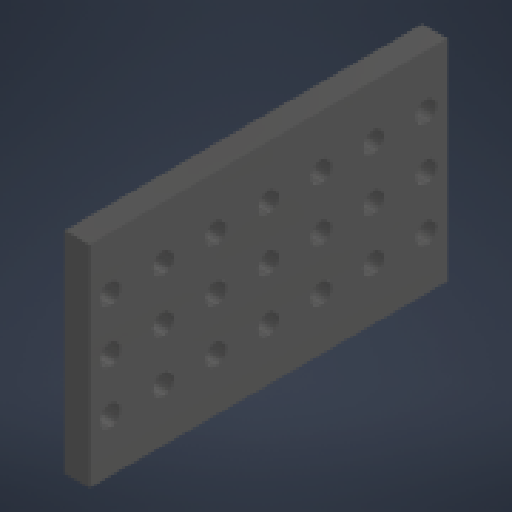
# Autodesk Inventor part: CHAPA FIXAÇÃO ESQUERDA 1
Saved by Autodesk Inventor 2026 (Build 300175000, 175)
## iProperties
Created: 2026-06-17
Part Number: CHAPA FIXAÇÃO ESQUERDA 1
Material: Genérico
Document SubType Name: Modeling
Designer: DELL
Density: 1 g/cm^3
Appearance: Cinza escuro
Author: DELL
Autodesk Inventor part; units mm, degrees
ref_plane "YZ Plane" through (0, 0, 0) normal (1, 0, 0) x (0, 1, 0)
ref_plane "XZ Plane" through (0, 0, 0) normal (0, 1, 0) x (-1, 0, 0)
ref_plane "XY Plane" through (0, 0, 0) normal (0, 0, 1) x (1, 0, 0)
sketch "Esboço1" plane through (0, 0, 0) normal (1, 0, 0) x (0, 1, 0)
  line L0 (0, 0) -> (50.8, 0)
  line L1 (50.8, 0) -> (50.8, -86.2)
  line L2 (50.8, -86.2) -> (0, -86.2)
  line L3 (0, -86.2) -> (0, 0)
  dimension "d0" = 50.8
  dimension "d1" = 86.2
  constraints: 8 end point, 2 parallel, 1 horizontal, 1 perpendicular
  measures "d0" distance of L1.end L2.end
  measures "d1" distance of L0.end L1.end
extrude "Extrusão1" add sketch "Esboço1" along normal blind 6
sketch "Esboço2" plane through (6, 0, 0) normal (1, 0, 0) x (0, 0, -1)
  circle A0 centre (5, 12.7) radius 2.5
  circle A1 centre (5, 25.4) radius 2.5
  circle A2 centre (5, 38.1) radius 2.5
  line L0 (0, 50.8) -> (0, 0) projected
  line L1 (86.2, 50.8) -> (0, 50.8) projected
  line L2 (0, 0) -> (86.2, 0) projected
  dimension "d4" = 5
  dimension "d5" = 5
  dimension "d6" = 5
  dimension "d7" = 5
  dimension "d8" = 5
  dimension "d9" = 5
  dimension "d10" = 12.7
  dimension "d11" = 12.7
  dimension "d12" = 12.7
  constraints: 3 centre point
  measures "d4" diameter of A0
  measures "d5" diameter of A1
  measures "d6" diameter of A2
  measures "d7" distance from line of L0 A0.centre
  measures "d8" distance from line of L0 A1.centre
  measures "d9" distance from line of L0 A2.centre
  measures "d10" distance from line of L1 A2.centre
  measures "d11" distance of A2.centre A1.centre
  measures "d12" distance of A1.centre A0.centre
extrude "Extrusão2" cut sketch "Esboço2" against normal blind 6
pattern_linear "Padrão retangular1" count 7 spacing 12.7 along (0, 0, -1) of "Extrusão2"
sketch "Esboço4" plane through (0, 0, 0) normal (-1, 0, 0) x (0, 0, 1)
  line L0 (-86.2, 0) -> (-86.2, 50.8) projected
  line L1 (-86.2, 50.8) -> (-162.4, 50.8)
  line L2 (-162.4, 50.8) -> (-162.4, 0)
  line L3 (-162.4, 0) -> (-86.2, 0)
  line L4 (-86.2, 0) -> (-86.2, 50.8)
  circle A0 centre (-157.4, 38.1) radius 2.5 projected
  circle A1 centre (-157.4, 25.4) radius 2.5 projected
  circle A2 centre (-157.4, 12.7) radius 2.5 projected
  circle A3 centre (-144.7, 12.7) radius 2.5 projected
  circle A4 centre (-144.7, 25.4) radius 2.5 projected
  circle A5 centre (-144.7, 38.1) radius 2.5 projected
  circle A6 centre (-132, 38.1) radius 2.5 projected
  circle A7 centre (-132, 25.4) radius 2.5 projected
  circle A8 centre (-132, 12.7) radius 2.5 projected
  line L5 (0, 0) -> (0, 50.8) projected
  line L6 (0, 50.8) -> (-467.2, 50.8) projected
  line L7 (-467.2, 50.8) -> (-467.2, 0) projected
  line L8 (0, 0) -> (-467.2, 0) projected
  circle A9 centre (-462.2, 12.7) radius 2.5 projected
  circle A10 centre (-462.2, 25.4) radius 2.5 projected
  circle A11 centre (-462.2, 38.1) radius 2.5 projected
  circle A12 centre (-449.5, 12.7) radius 2.5 projected
  circle A13 centre (-449.5, 25.4) radius 2.5 projected
  circle A14 centre (-449.5, 38.1) radius 2.5 projected
  circle A15 centre (-436.8, 12.7) radius 2.5 projected
  circle A16 centre (-436.8, 25.4) radius 2.5 projected
  circle A17 centre (-436.8, 38.1) radius 2.5 projected
  circle A18 centre (-424.1, 12.7) radius 2.5 projected
  circle A19 centre (-424.1, 25.4) radius 2.5 projected
  circle A20 centre (-424.1, 38.1) radius 2.5 projected
  circle A21 centre (-411.4, 12.7) radius 2.5 projected
  circle A22 centre (-411.4, 25.4) radius 2.5 projected
  circle A23 centre (-411.4, 38.1) radius 2.5 projected
  circle A24 centre (-398.7, 12.7) radius 2.5 projected
  circle A25 centre (-398.7, 25.4) radius 2.5 projected
  circle A26 centre (-398.7, 38.1) radius 2.5 projected
  circle A27 centre (-386, 12.7) radius 2.5 projected
  circle A28 centre (-386, 25.4) radius 2.5 projected
  circle A29 centre (-386, 38.1) radius 2.5 projected
  circle A30 centre (-373.3, 12.7) radius 2.5 projected
  circle A31 centre (-373.3, 25.4) radius 2.5 projected
  circle A32 centre (-373.3, 38.1) radius 2.5 projected
  circle A33 centre (-360.6, 12.7) radius 2.5 projected
  circle A34 centre (-360.6, 25.4) radius 2.5 projected
  circle A35 centre (-360.6, 38.1) radius 2.5 projected
  circle A36 centre (-347.9, 12.7) radius 2.5 projected
  circle A37 centre (-347.9, 25.4) radius 2.5 projected
  circle A38 centre (-347.9, 38.1) radius 2.5 projected
  circle A39 centre (-335.2, 12.7) radius 2.5 projected
  circle A40 centre (-335.2, 25.4) radius 2.5 projected
  circle A41 centre (-335.2, 38.1) radius 2.5 projected
  circle A42 centre (-322.5, 12.7) radius 2.5 projected
  circle A43 centre (-322.5, 25.4) radius 2.5 projected
  circle A44 centre (-322.5, 38.1) radius 2.5 projected
  circle A45 centre (-309.8, 12.7) radius 2.5 projected
  circle A46 centre (-309.8, 25.4) radius 2.5 projected
  circle A47 centre (-309.8, 38.1) radius 2.5 projected
  circle A48 centre (-297.1, 12.7) radius 2.5 projected
  circle A49 centre (-297.1, 25.4) radius 2.5 projected
  circle A50 centre (-297.1, 38.1) radius 2.5 projected
  circle A51 centre (-284.4, 12.7) radius 2.5 projected
  circle A52 centre (-284.4, 25.4) radius 2.5 projected
  circle A53 centre (-284.4, 38.1) radius 2.5 projected
  circle A54 centre (-271.7, 12.7) radius 2.5 projected
  circle A55 centre (-271.7, 25.4) radius 2.5 projected
  circle A56 centre (-271.7, 38.1) radius 2.5 projected
  circle A57 centre (-259, 12.7) radius 2.5 projected
  circle A58 centre (-259, 25.4) radius 2.5 projected
  circle A59 centre (-259, 38.1) radius 2.5 projected
  circle A60 centre (-246.3, 12.7) radius 2.5 projected
  circle A61 centre (-246.3, 25.4) radius 2.5 projected
  circle A62 centre (-246.3, 38.1) radius 2.5 projected
  circle A63 centre (-233.6, 12.7) radius 2.5 projected
  circle A64 centre (-233.6, 25.4) radius 2.5 projected
  circle A65 centre (-233.6, 38.1) radius 2.5 projected
  circle A66 centre (-220.9, 12.7) radius 2.5 projected
  circle A67 centre (-220.9, 25.4) radius 2.5 projected
  circle A68 centre (-220.9, 38.1) radius 2.5 projected
  circle A69 centre (-208.2, 12.7) radius 2.5 projected
  circle A70 centre (-208.2, 25.4) radius 2.5 projected
  circle A71 centre (-208.2, 38.1) radius 2.5 projected
  circle A72 centre (-195.5, 12.7) radius 2.5 projected
  circle A73 centre (-195.5, 25.4) radius 2.5 projected
  circle A74 centre (-195.5, 38.1) radius 2.5 projected
  circle A75 centre (-182.8, 12.7) radius 2.5 projected
  circle A76 centre (-182.8, 25.4) radius 2.5 projected
  circle A77 centre (-182.8, 38.1) radius 2.5 projected
  circle A78 centre (-170.1, 12.7) radius 2.5 projected
  circle A79 centre (-170.1, 25.4) radius 2.5 projected
  circle A80 centre (-170.1, 38.1) radius 2.5 projected
  circle A81 centre (-157.4, 12.7) radius 2.5 projected
  circle A82 centre (-157.4, 25.4) radius 2.5 projected
  circle A83 centre (-157.4, 38.1) radius 2.5 projected
  circle A84 centre (-144.7, 12.7) radius 2.5 projected
  circle A85 centre (-144.7, 25.4) radius 2.5 projected
  circle A86 centre (-144.7, 38.1) radius 2.5 projected
  circle A87 centre (-132, 12.7) radius 2.5 projected
  circle A88 centre (-132, 25.4) radius 2.5 projected
  circle A89 centre (-132, 38.1) radius 2.5 projected
  circle A90 centre (-119.3, 12.7) radius 2.5 projected
  circle A91 centre (-119.3, 25.4) radius 2.5 projected
  circle A92 centre (-119.3, 38.1) radius 2.5 projected
  circle A93 centre (-106.6, 12.7) radius 2.5 projected
  circle A94 centre (-106.6, 25.4) radius 2.5 projected
  circle A95 centre (-106.6, 38.1) radius 2.5 projected
  circle A96 centre (-93.9, 12.7) radius 2.5 projected
  circle A97 centre (-93.9, 25.4) radius 2.5 projected
  circle A98 centre (-93.9, 38.1) radius 2.5 projected
  circle A99 centre (-81.2, 12.7) radius 2.5 projected
  circle A100 centre (-81.2, 25.4) radius 2.5 projected
  circle A101 centre (-81.2, 38.1) radius 2.5 projected
  circle A102 centre (-68.5, 12.7) radius 2.5 projected
  circle A103 centre (-68.5, 25.4) radius 2.5 projected
  circle A104 centre (-68.5, 38.1) radius 2.5 projected
  circle A105 centre (-55.8, 12.7) radius 2.5 projected
  circle A106 centre (-55.8, 25.4) radius 2.5 projected
  circle A107 centre (-55.8, 38.1) radius 2.5 projected
  circle A108 centre (-43.1, 12.7) radius 2.5 projected
  circle A109 centre (-43.1, 25.4) radius 2.5 projected
  circle A110 centre (-43.1, 38.1) radius 2.5 projected
  circle A111 centre (-30.4, 12.7) radius 2.5 projected
  circle A112 centre (-30.4, 25.4) radius 2.5 projected
  circle A113 centre (-30.4, 38.1) radius 2.5 projected
  circle A114 centre (-17.7, 12.7) radius 2.5 projected
  circle A115 centre (-17.7, 25.4) radius 2.5 projected
  circle A116 centre (-17.7, 38.1) radius 2.5 projected
  circle A117 centre (-5, 12.7) radius 2.5 projected
  circle A118 centre (-5, 25.4) radius 2.5 projected
  circle A119 centre (-5, 38.1) radius 2.5 projected
  dimension "d19" = 5
  constraints: 8 end point, 2 parallel, 1 horizontal, 1 perpendicular
  measures "d19" distance from line of L2 A0.centre
extrude "Extrusão3" add sketch "Esboço4" against normal blind 6 contours L3 L2 L1 L0
equation "\"d8\" = d7"
equation "\"d9\" = d8"
equation "\"d11\" = d10"
equation "\"d12\" = d11"
